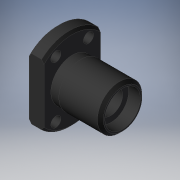
# Autodesk Inventor part: MDK 0802-30420 Nut
Saved by Autodesk Inventor 2019 (Build 230136000, 136)
## iProperties
Created: 2024-04-08
Part Number: MDK 0802-30420 Nut
Material: Generic
Catalog Web Link: www.cadenas.de
Description: Miniature non-preloaded type MDK-Nut-
Vendor: THK
Document SubType Name: Modeling
Designer: psAdmin
Manufacturer: THK
Mass: 3.56186 g
Surface Area: 28.3567 cm^2
Volume: 3.56186 cm^3
Density: 1 g/cm^3
Appearance: PSOLRGB-175-175-175
Category: PARTsolutions
Company: THK
Title: MDK 0802-30420 Nut
Author: Cadenas PARTsolutions
PSOL_IDENT_0: {$CADENAS_DATA/23d-libs/thk/fed_screw/ball_screw/ball_screw/standard_lead_prec_gbs/miniature_mdk_2.p
PSOL_IDENT_1: rj},225 {VTYP=3D},{NB=MDK 0802-30420 Nut},{LINA=MDK 0802-30420 Nut},{NN=Miniature non-preloaded type
PSOL_IDENT_2: MDK-Nut},{DATE=01.04.2024 00:21:36},{GEOMDATE=28.04.2017 07:45:12},{VERSION=},{LINEID=50},{WBVAR=ST
PSOL_IDENT_3: ,FS,SS,PN,TS},{WBNUMERIC=ST,PN}  {NB=MDK 0802-30420 Nut},{LINA=MDK 0802-30420 Nut},{KT=DUMMY},{IDNR=
PSOL_IDENT_4: },{TP=MDK series},{MN=MDK 0802-3},{ST=0.0},{STX=278},{NOTE1=There is the groove on both ends of the
PSOL_IDENT_5: stroke},{FS=},{FSX='','None','H1','Type_H1','H3','Type_H3'},{SS=},{OL=42},{NOTE2=Overall thread leng
PSOL_IDENT_6: th is added to the both ends},{PN=0},{PNX=0},{SS1='','None'},{TS=},{TSX='','None'},{OLX=42},{OL3=0},
PSOL_IDENT_7: {OL4=0},{D=8},{EL=290.000},{L=22.000},{E2=0.000},{E=30.000},{F=8.000},{E1=0.000},{F1=0.000},{N=4.000
PSOL_IDENT_8: },{H=4.000},{ELX=22},{FSXX=},{SS2=},{PITCH=1.250},{LN=5.000},{A2=5.000},{B=4.000},{S2=7.000},{J=5.00
PSOL_IDENT_9: 0},{G=0.000},{T=0.000},{P=5.000},{R=3.700},{PITCH3=0.500},{OD=15.000},{FD=28.000},{H1=5.000},{B1=17.
PSOL_IDENT_10: 000},{PCD=22.000},{SD1=3.400},{TW=19.000},{PCD1=17.320},{D2=12.000}
NB: MDK 0802-30420 Nut
NN: Miniature non-preloaded type MDK-Nut
NBSYN: $MN.$TS.$ST.$FS.$SS.$OL.$PN. Nut
LINA: MDK 0802-30420 Nut
CATALOG: THK
TP: MDK series
MN: MDK 0802-3
ST: 0
NOTE1: There is the groove on both ends of the stroke
NOTE2: Overall thread length is added to the both ends
PN: 0
D: 8
EL: 290
L: 22
E2: 0
E: 30
F: 8
E1: 0
F1: 0
N: 4
H: 4
PITCH: 1.25
LN: 5
A2: 5
B: 4
S2: 7
J: 5
G: 0
T: 0
P: 5
R: 3.7
PITCH3: 0.5
OD: 15
FD: 28
H1: 5
B1: 17
PCD: 22
SD1: 3.4
TW: 19
PCD1: 17.32
D2: 12
SUPPLIER: THK
ARTICLENO: MDK 0802-30420 Nut
BOMINFO: MDK 0802-30420 Nut
CREATOR: CADENAS GmbH
Autodesk Inventor part; units mm, degrees
sketch "Sketch_1" plane through (0, 0, 0) normal (1, 0, 0) x (0, 1, 0)
  line L0 (10.2835, 9.5) -> (-10.2835, 9.5)
  arc A0 (-10.2835, 9.5) -> (-10.2835, -9.5) centre (0, 0) ccw
  line L1 (-10.2835, -9.5) -> (10.2835, -9.5)
  arc A1 (10.2835, -9.5) -> (10.2835, 9.5) centre (0, 0) ccw
  constraints: 4 end point, 4 point on circle, 2 centre point
extrude "Extrusion1" add sketch "Sketch_1" along normal blind 5
sketch "Sketch_9" plane through (0, 0, 0) normal (0, 0, 1) x (1, 0, 0)
  line L0 (50, 0) -> (-50, 0)
  line L1 (0, 13.2) -> (1, 14.2)
  line L2 (1, 14.2) -> (0, 14.2)
  line L3 (0, 14.2) -> (0, 13.2)
  constraints: 8 end point
revolve "Revolution1" cut sketch "Sketch_9" angle 360 about axis through (50, 0, 0) along (1, 0, 0)
sketch "Sketch_10" plane through (0, 0, 0) normal (0, 0, 1) x (1, 0, 0)
  line L0 (50, 0) -> (-50, 0)
  line L1 (4, 14.2) -> (5, 13.2)
  line L2 (5, 13.2) -> (5, 14.2)
  line L3 (5, 14.2) -> (4, 14.2)
  constraints: 8 end point
revolve "Revolution2" cut sketch "Sketch_10" angle 360 about axis through (50, 0, 0) along (1, 0, 0)
sketch "Sketch4" plane through (5, 0, 0) normal (1, 0, 0) x (0, 0, -1)
  point P0 (-5.5, 9.5263)
hole "Hole1" at (5, 9.5263, 5.5) direction (-1, 0, 0) diameter 3.4 depth 5
sketch "Sketch5" plane through (5, 0, 0) normal (1, 0, 0) x (0, 0, -1)
  point P0 (5.5, -9.5263)
hole "Hole2" at (5, -9.5263, -5.5) direction (-1, 0, 0) diameter 3.4 depth 5
sketch "Sketch6" plane through (5, 0, 0) normal (1, 0, 0) x (0, 0, -1)
  point P0 (5.5, 9.5263)
hole "Hole3" at (5, 9.5263, -5.5) direction (-1, 0, 0) diameter 3.4 depth 5
sketch "Sketch7" plane through (5, 0, 0) normal (1, 0, 0) x (0, 0, -1)
  point P0 (-5.5, -9.5263)
hole "Hole4" at (5, -9.5263, 5.5) direction (-1, 0, 0) diameter 3.4 depth 5
sketch "Sketch8" plane through (0, 0, 0) normal (-1, 0, 0) x (0, 0, 1)
  point P0 (0, 0)
hole "Hole5" at (0, 0, 0) direction (1, 0, 0) diameter 8 depth 5
sketch "Sketch_14" plane through (0, 0, 0) normal (0, 0, 1) x (1, 0, 0)
  line L0 (50, 0) -> (-50, 0)
  line L1 (5, 7.2) -> (5, 4)
  line L2 (5, 4) -> (22, 4)
  line L3 (22, 4) -> (22, 6.5)
  line L4 (22, 6.5) -> (21, 7.5)
  line L5 (21, 7.5) -> (8, 7.5)
  line L6 (8, 7.5) -> (8, 7.2)
  line L7 (8, 7.2) -> (5, 7.2)
  constraints: 16 end point
revolve "Revolution3" add sketch "Sketch_14" angle 360 about axis through (50, 0, 0) along (1, 0, 0)
sketch "Sketch_5" plane through (0, 0, 0) normal (1, 0, 0) x (0, 1, 0)
  circle A0 centre (0, 0) radius 6
  constraints: 1 centre point
extrude "Extrusion2" cut sketch "Sketch_5" along normal blind 4
sketch "Sketch_6" plane through (22, 0, 0) normal (1, 0, 0) x (0, 0, -1)
  circle A0 centre (0, 0) radius 6
  constraints: 1 centre point
extrude "Extrusion3" cut sketch "Sketch_6" against normal blind 4
ref_plane "mdk_2_XY" through (0, 0, 0) normal (1, 0, 0) x (0, 0, -1)
ref_plane "mdk_2_YZ" through (0, 0, 0) normal (0, 0, -1) x (0, 1, 0)
ref_plane "mdk_2_ZX" through (0, 0, 0) normal (0, 1, 0) x (1, 0, 0)
body "Solid1"
